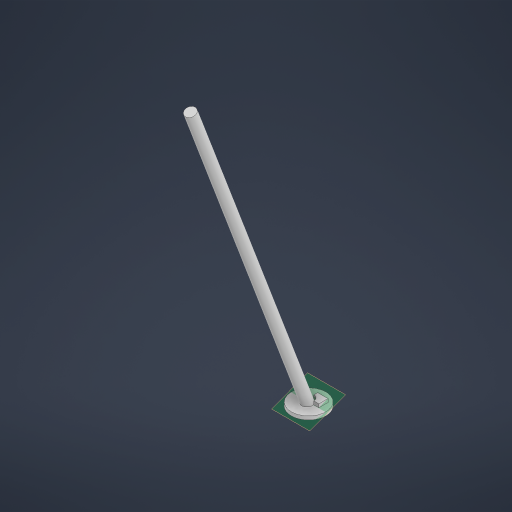
# Autodesk Inventor part: Legs
Saved by Autodesk Inventor 2023.2 (Build 272271030, 271C)
## iProperties
Created: 2023-04-10
Part Number: Legs
Material: Generic
Document SubType Name: Modeling
Designer: ckeer
Density: 1 g/cm^3
Appearance: Default
Author: ckeer
Autodesk Inventor part; units mm, degrees
ref_plane "YZ Plane" through (0, 0, 0) normal (1, 0, 0) x (0, 1, 0)
ref_plane "XZ Plane" through (0, 0, 0) normal (0, 1, 0) x (-1, 0, 0)
ref_plane "XY Plane" through (0, 0, 0) normal (0, 0, 1) x (1, 0, 0)
sketch "Sketch1" plane through (0, 0, 0) normal (0, 1, 0) x (-1, 0, 0)
  circle A0 centre (0, 0) radius 63.5
  dimension "d0" = 127
  constraints: 1 centre point, 1 coincident
  measures "d0" diameter of A0
extrude "Extrusion1" add sketch "Sketch1" along normal blind 12.7
sketch "Sketch2" plane through (0, 12.7, 0) normal (0, 1, 0) x (1, 0, 0)
  circle A0 centre (0, 0) radius 19.05
  circle A1 centre (0, 0) radius 63.5 projected
  line L0 (0, 0) -> (37.7183, 0)
  line L1 (37.7183, 0) -> (37.7183, 33.6732)
  line L2 (37.7183, 33.6732) -> (0, 33.6732)
  line L3 (0, 33.6732) -> (0, 0)
  point P0 (63.5, 0)
  point P1 (0, 19.05)
  point P2 (19.05, 0)
  dimension "d3" = 38.1
  constraints: 8 end point, 2 parallel, 1 centre point, 1 coincident, 1 horizontal, 1 horizontal alignment, 1 perpendicular, 1 other
  measures "d3" diameter of A0
extrude "Extrusion2" add sketch "Sketch2" along normal blind 12.7 contours A0 L3 L2 L1 L0
ref_plane "Work Plane1" through (9.525, 12.7, 0) normal (0, -0.9356646, -0.3528907) x (-1, 0, 0)
sketch "Sketch3" plane through (9.525, 12.7, 0) normal (0, -0.9356646, -0.3528907) x (-1, 0, 0)
  circle A0 centre (9.525, -4.4817) radius 19.05
  dimension "d6" = 38.1
  constraints: 1 centre point, 1 coincident
  measures "d6" diameter of A0
extrude "Extrusion3" add sketch "Sketch3" along normal blind 4.826
sketch "Sketch4" plane through (9.525, 12.7, 0) normal (0, 0.9356646, 0.3528907) x (1, 0, 0)
  circle A0 centre (-9.525, -4.4817) radius 19.05
  constraints: 1 centre point, 1 coincident
extrude "Extrusion4" add sketch "Sketch4" along normal blind 1219.2
body "Solid1"
